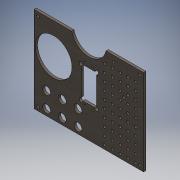
# Autodesk Inventor part: A0001
Saved by Autodesk Inventor 2017 (Build 210142000, 142)
## iProperties
Part Number: A0001
Material: ABS 塑膠
Document SubType Name: Modeling
Designer: lygfy
Density: 1.06 g/cm^3
Appearance: 胡桃木
Author: lygfy
Autodesk Inventor part; units mm, degrees
ref_plane "YZ Plane" through (0, 0, 0) normal (1, 0, 0) x (0, 1, 0)
ref_plane "XZ Plane" through (0, 0, 0) normal (0, 1, 0) x (-1, 0, 0)
ref_plane "XY Plane" through (0, 0, 0) normal (0, 0, 1) x (1, 0, 0)
sketch "草圖1" plane through (0, 0, 0) normal (0, 1, 0) x (-1, 0, 0)
  line L0 (7.5, -20) -> (-7.5, -20)
  line L1 (-10, -17.5) -> (-10, 17.5)
  line L2 (-7.5, 20) -> (7.5, 20)
  line L3 (10, 17.5) -> (10, -17.5)
  line L4 (70, 50) -> (70, -60)
  line L5 (70, -60) -> (-70, -60)
  line L6 (-70, -60) -> (-70, 50)
  arc A0 (-7.5, 20) -> (-10, 17.5) centre (-10, 20) ccw
  arc A1 (10, 17.5) -> (7.5, 20) centre (10, 20) ccw
  arc A2 (7.5, -20) -> (10, -17.5) centre (10, -20) ccw
  arc A3 (-10, -17.5) -> (-7.5, -20) centre (-10, -20) ccw
  arc A4 (-21.9374, 50) -> (21.9374, 50) centre (0, 55) ccw
  line L7 (-70, 50) -> (-21.9374, 50)
  line L8 (21.9374, 50) -> (70, 50)
  point P0 (0, 0)
  point P1 (-10, 0)
  point P2 (0, 20)
  point P3 (-10, 0)
  point P4 (0, -60)
  dimension "d2" = 5
  dimension "d3" = 40
  dimension "d4" = 20
  dimension "d19" = 45
  dimension "d20" = 55
  dimension "d21" = 140
  dimension "d30" = 110
  dimension "d31" = 60
  constraints: 18 end point, 10 point on circle, 8 point on line, 5 centre point, 4 midpoint, 3 equal radius, 3 horizontal, 3 parallel, 3 vertical alignment, 2 horizontal alignment, 2 vertical, 1 collinear, 1 perpendicular
  measures "d2" diameter of A0
  measures "d3" distance between parallel lines of L0 L2
  measures "d4" distance between parallel lines of L1 L3
  measures "d19" diameter of A4
  measures "d20" distance of point (0, 0) A4.centre
  measures "d21" distance of L4.end L5.end
  measures "d30" distance of L4.start L4.end
  measures "d31" distance from line of L5 point (0, 0)
extrude "擠出1" add sketch "草圖1" along normal mid plane 3
sketch "草圖4" plane through (0, -1.5, 0) normal (0, -1, 0) x (1, 0, 0)
  line L0 (-65, 45) -> (65, 45)
  line L1 (65, 45) -> (65, -55)
  line L2 (65, -55) -> (-65, -55)
  line L3 (-65, -55) -> (-65, 45)
  line L4 (70, -60) -> (70, 50) projected
  line L5 (-21.9374, 50) -> (-70, 50) projected
  point P0 (0, 0)
  point P1 (0, -55)
  dimension "d32" = 5
  dimension "d34" = 5
  dimension "d35" = 5
  constraints: 8 end point, 2 parallel, 1 horizontal, 1 midpoint, 1 perpendicular, 1 vertical alignment
  measures "d32" distance between parallel lines of L1 L4
  measures "d34" distance between parallel lines of L0 L5
  measures "d35" distance from line of L4.start L2
hole "孔3" at (-65, -1.5, 45) at (-65, -1.5, -55) at (65, -1.5, 45) at (65, -1.5, -55) direction (0, 1, 0) diameter 3.2 end through all
sketch "草圖2" plane through (0, -1.5, 0) normal (0, -1, 0) x (1, 0, 0)
  line L0 (-5, 24) -> (5, 24)
  line L1 (5, 24) -> (5, -24)
  line L2 (5, -24) -> (-5, -24)
  line L3 (-5, -24) -> (-5, 24)
  point P0 (0, 0)
  point P1 (5, 0)
  point P2 (0, 24)
  dimension "d9" = 10
  dimension "d10" = 48
  constraints: 8 end point, 2 midpoint, 2 parallel, 1 horizontal, 1 horizontal alignment, 1 perpendicular, 1 vertical alignment
  measures "d9" distance of L1.end L2.end
  measures "d10" distance of L0.end L1.end
hole "孔1" at (-5, -1.5, 24) at (5, -1.5, 24) at (5, -1.5, -24) at (-5, -1.5, -24) direction (0, 1, 0) diameter 2.459 depth 8.8 tip angle 118 thread size "M3x0.5" class "6H" standard "ISO Metric profile"
sketch "草圖3" plane through (0, -1.5, 0) normal (0, -1, 0) x (1, 0, 0)
  arc A0 (0, 77.5) -> (0, 32.5) centre (0, 55) ccw projected
  point P0 (45, 10)
  point P1 (31.3889, 42.245)
hole "孔2" at (31.3889, -1.5, 42.245) at (45, -1.5, 10) direction (0, 1, 0) diameter 3.2 end through all
sketch "草圖5" plane through (0, -1.5, 0) normal (0, -1, 0) x (1, 0, 0)
  circle A0 centre (-45, 10) radius 23.5 projected
  point P0 (0, 0)
extrude "擠出2" cut sketch "草圖5" along normal through all both and the other way through all
sketch "草圖6" plane through (0, 0, 0) normal (0, 1, 0) x (-1, 0, 0)
  circle A0 centre (54, -52) radius 5
  line L0 (98, 0) -> (-98, 0) construction
  line L1 (0, -82) -> (0, 72) construction
  circle A1 centre (54, -32) radius 5
  circle A2 centre (34, -52) radius 5
  circle A3 centre (34, -32) radius 5
  circle A4 centre (14, -52) radius 5
  circle A5 centre (14, -32) radius 5
  circle A6 centre (-20, -55) radius 1.6
  circle A7 centre (-20, -45) radius 1.6
  circle A8 centre (-20, -35) radius 1.6
  circle A9 centre (-20, -25) radius 1.6
  circle A10 centre (-20, -15) radius 1.6
  circle A11 centre (-30, -55) radius 1.6
  circle A12 centre (-30, -45) radius 1.6
  circle A13 centre (-30, -35) radius 1.6
  circle A14 centre (-30, -25) radius 1.6
  circle A15 centre (-30, -15) radius 1.6
  circle A16 centre (-40, -55) radius 1.6
  circle A17 centre (-40, -45) radius 1.6
  circle A18 centre (-40, -35) radius 1.6
  circle A19 centre (-40, -25) radius 1.6
  circle A20 centre (-40, -15) radius 1.6
  circle A21 centre (-50, -55) radius 1.6
  circle A22 centre (-50, -45) radius 1.6
  circle A23 centre (-50, -35) radius 1.6
  circle A24 centre (-50, -25) radius 1.6
  circle A25 centre (-50, -15) radius 1.6
  circle A26 centre (-60, -55) radius 1.6
  circle A27 centre (-60, -45) radius 1.6
  circle A28 centre (-60, -35) radius 1.6
  circle A29 centre (-60, -25) radius 1.6
  circle A30 centre (-60, -15) radius 1.6
  circle A31 centre (-20, -5) radius 1.6
  circle A32 centre (-30, -5) radius 1.6
  circle A33 centre (-40, -5) radius 1.6
  circle A34 centre (-50, -5) radius 1.6
  circle A35 centre (-60, -5) radius 1.6
  circle A36 centre (-20, 5) radius 1.6
  circle A37 centre (-30, 5) radius 1.6
  circle A38 centre (-40, 5) radius 1.6
  circle A39 centre (-50, 5) radius 1.6
  circle A40 centre (-60, 5) radius 1.6
  circle A41 centre (-20, 15) radius 1.6
  circle A42 centre (-30, 15) radius 1.6
  circle A43 centre (-40, 15) radius 1.6
  circle A44 centre (-50, 15) radius 1.6
  circle A45 centre (-60, 15) radius 1.6
  circle A46 centre (-20, 25) radius 1.6
  circle A47 centre (-30, 25) radius 1.6
  circle A48 centre (-40, 25) radius 1.6
  circle A49 centre (-50, 25) radius 1.6
  circle A50 centre (-60, 25) radius 1.6
  circle A51 centre (-20, 35) radius 1.6
  circle A52 centre (-30, 35) radius 1.6
  circle A53 centre (-40, 35) radius 1.6
  circle A54 centre (-50, 35) radius 1.6
  circle A55 centre (-60, 35) radius 1.6
  line L2 (70, 50) -> (70, -60) projected
  line L3 (70, -60) -> (-70, -60) projected
  line L4 (-70, -60) -> (-70, 50) projected
  point P0 (0, 0)
  dimension "d45" = 10
  dimension "d48" = 20
  dimension "d51" = 20
  dimension "d54" = 3.2
  dimension "d57" = 10
  dimension "d60" = 10
  dimension "d65" = 16
  dimension "d66" = 8
  dimension "d67" = 5
  dimension "d68" = 50
  constraints: 56 centre point, 2 horizontal, 2 vertical, 108 other
  measures "d45" diameter of A0
  measures "d48" distance of A0.centre A1.centre
  measures "d51" distance of A0.centre A2.centre
  measures "d54" diameter of A6
  measures "d57" distance of A6.centre A7.centre
  measures "d60" distance of A6.centre A11.centre
  measures "d65" distance from line of A0.centre L2
  measures "d66" distance from line of L3 A0.centre
  measures "d67" distance from line of A6.centre L3
  measures "d68" distance from line of L4 A6.centre
extrude "擠出3" cut sketch "草圖6" along normal through all both and the other way through all
equation "\"d34\" = d33"
equation "\"d35\" = d32"
equation "\"d33\" = 5"
